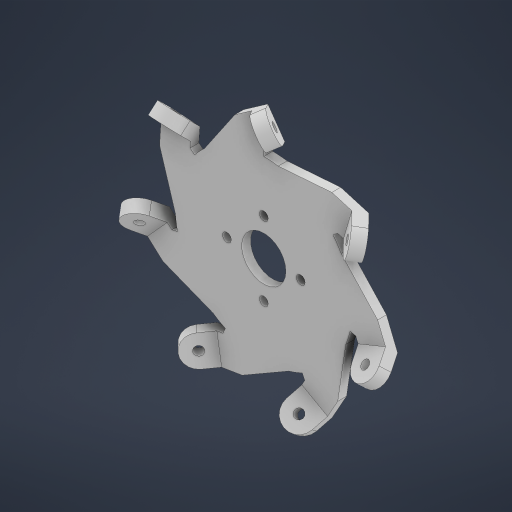
# Autodesk Inventor part: Outer plate
Saved by Autodesk Inventor 2023 (Build 270158000, 158)
## iProperties
Created: 2023-04-05
Part Number: Outer plate
Material: Generic
Document SubType Name: Modeling
Designer: vatdu
Density: 1 g/cm^3
Appearance: Default
Author: vatdu
Autodesk Inventor part; units mm, degrees
ref_plane "YZ Plane" through (0, 0, 0) normal (1, 0, 0) x (0, 1, 0)
ref_plane "XZ Plane" through (0, 0, 0) normal (0, 1, 0) x (-1, 0, 0)
sketch "Sketch1" plane through (0, 0, 0) normal (0, 0, 1) x (1, 0, 0)
  circle A0 centre (0, 0) radius 30
  circle A1 centre (0, 0) radius 7.5
  line L0 (0, 30) -> (0, 32)
  line L1 (0, 32) -> (4.0958, 34.8679)
  line L2 (0, 32) -> (5, 32) construction
  line L3 (4.0958, 34.8679) -> (-1.64, 43.0594)
  line L4 (-1.64, 43.0594) -> (-9.8315, 37.3236)
  line L5 (-9.8315, 37.3236) -> (-20.1018, 22.2692)
  line L6 (-35.3107, 15.5843) -> (-29.944, -1.8316)
  line L7 (-34.6877, 25.5649) -> (-35.3107, 15.5843)
  line L8 (-24.7071, 24.942) -> (-34.6877, 25.5649)
  line L9 (-25.0186, 19.9517) -> (-24.7071, 24.942)
  line L10 (-23.4549, 18.7047) -> (-25.0186, 19.9517)
  line L11 (-34.2001, -17.8903) -> (-17.2378, -24.5532)
  line L12 (-41.6149, -11.1805) -> (-34.2001, -17.8903)
  line L13 (-34.9051, -3.7658) -> (-41.6149, -11.1805)
  line L14 (-31.1977, -7.1207) -> (-34.9051, -3.7658)
  line L15 (-29.2478, -6.6756) -> (-31.1977, -7.1207)
  line L16 (-7.3362, -37.8932) -> (8.4488, -28.7857)
  line L17 (-17.2052, -39.5068) -> (-7.3362, -37.8932)
  line L18 (-18.8188, -29.6378) -> (-17.2052, -39.5068)
  line L19 (-13.8843, -28.831) -> (-18.8188, -29.6378)
  line L20 (-13.0165, -27.0291) -> (-13.8843, -28.831)
  line L21 (25.052, -29.3617) -> (27.7733, -11.342)
  line L22 (20.1604, -38.0836) -> (25.052, -29.3617)
  line L23 (11.4385, -33.192) -> (20.1604, -38.0836)
  line L24 (13.8843, -28.831) -> (11.4385, -33.192)
  line L25 (13.0165, -27.0291) -> (13.8843, -28.831)
  line L26 (38.5756, 1.2797) -> (26.1839, 14.6424)
  line L27 (42.3447, -7.9827) -> (38.5756, 1.2797)
  line L28 (33.0823, -11.7519) -> (42.3447, -7.9827)
  line L29 (31.1977, -7.1207) -> (33.0823, -11.7519)
  line L30 (29.2478, -6.6756) -> (31.1977, -7.1207)
  line L31 (23.0509, 30.9575) -> (4.8775, 29.6008)
  line L32 (32.6427, 28.1293) -> (23.0509, 30.9575)
  line L33 (29.8145, 18.5376) -> (32.6427, 28.1293)
  line L34 (25.0186, 19.9517) -> (29.8145, 18.5376)
  line L35 (23.4549, 18.7047) -> (25.0186, 19.9517)
  circle A2 centre (-12.5, 0) radius 1.5
  circle A3 centre (0, 12.5) radius 1.5
  circle A4 centre (12.5, 0) radius 1.5
  circle A5 centre (0, -12.5) radius 1.5
  dimension "d1" = 15
  dimension "d2" = 2
  dimension "d4" = 5
  dimension "d5" = 35
  dimension "d6" = 10
  dimension "d7" = 10
  dimension "d10" = 360
  dimension "d28" = 3
  dimension "d29" = 3
  dimension "d30" = 3
  dimension "d31" = 3
  constraints: 72 end point, 6 centre point, 2 coincident, 2 perpendicular, 2 point on circle, 1 equal length, 1 horizontal, 1 vertical, 78 other
  measures "d1" diameter of A1
  measures "d2" distance of L0.start L0.end
  measures "d4" distance of L0.end L1.end
  measures "d5" angle of L2 L1
  measures "d6" distance of L1.end L3.end
  measures "d7" distance of L3.end L4.end
  measures "d28" diameter of A2
  measures "d29" diameter of A3
  measures "d30" diameter of A4
  measures "d31" diameter of A5
extrude "Extrusion1" add sketch "Sketch1" along normal blind 3
ref_plane "Work Plane1" through (33.0823, -11.7519, 0) normal (-0.2665207, 0.6549555, -0.7071068) x (0.926247, 0.3769172, 0)
sketch "Sketch2" plane through (33.0823, -11.7519, 0) normal (-0.2665207, 0.6549555, -0.7071068) x (0.926247, 0.3769172, 0)
  line L0 (0, 0) -> (10, 0) projected
  line L1 (10, -2.1213) -> (10, -9.1924) projected
  line L2 (0, 0) -> (10, 0)
  line L3 (10, 0) -> (10, -4.1952)
  line L4 (10, -4.1952) -> (0, -4.1952)
  line L5 (0, -4.1952) -> (0, 0)
  point P0 (-26.2129, -16.5141)
  point P1 (10, -2.1213)
  point P2 (10, 0)
  constraints: 8 end point, 2 parallel, 1 horizontal, 1 perpendicular, 1 point on line
extrude "Extrusion2" add sketch "Sketch2" against normal blind 10
fillet "Fillet1" radius 5 2 edges at (44.4509, -13.1585, 8.5543) (35.1884, -16.9276, 8.5543)
sketch "Sketch3" plane through (31.9768, -9.0353, 3) normal (-0.2665207, 0.6549555, 0.7071068) x (0.926247, 0.3769172, 0)
  line L0 (10, 0.0475) -> (10, -4.9525) projected
  line L1 (10, -4.9525) -> (-0.1243, -4.9525)
  circle A0 centre (4.9378, -4.9525) radius 1.5
  point P0 (-26.2129, 16.5615)
  dimension "d18" = 3
  constraints: 2 end point, 1 centre point, 1 horizontal, 1 midpoint
  measures "d18" diameter of A0
extrude "Extrusion3" cut sketch "Sketch3" against normal blind 10
pattern_circular "Circular Pattern1" count 7 over 360 about axis through (0, 0, 0) along (0, 0, 1) of "Extrusion2"
pattern_circular "Circular Pattern2" count 7 over 360 about axis through (0, 0, 0) along (0, 0, 1) of "Fillet1", "Extrusion3"
body "Solid1"
